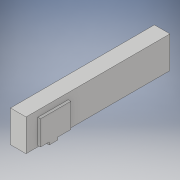
# Autodesk Inventor part: Nerf Gun
Saved by Autodesk Inventor 2018 (Build 220112000, 112)
## iProperties
Created: 2018-11-04
Part Number: Nerf Gun
Material: Generic
Document SubType Name: Modeling
Designer: Cameron
Density: 1 g/cm^3
Appearance: Default
Author: Cameron
Autodesk Inventor part; units mm, degrees
ref_plane "YZ Plane" through (0, 0, 0) normal (1, 0, 0) x (0, 1, 0)
ref_plane "XZ Plane" through (0, 0, 0) normal (0, 1, 0) x (-1, 0, 0)
ref_plane "XY Plane" through (0, 0, 0) normal (0, 0, 1) x (1, 0, 0)
sketch "Sketch1" plane through (0, 0, 0) normal (1, 0, 0) x (0, 1, 0)
  line L0 (42.5, 52.75) -> (-42.5, 52.75)
  line L1 (-42.5, 52.75) -> (-42.5, -52.75)
  line L2 (-42.5, -52.75) -> (42.5, -52.75)
  line L3 (42.5, -52.75) -> (42.5, 52.75)
  line L4 (-42.5, 22.75) -> (-51.5, 22.75)
  line L5 (-51.5, 22.75) -> (-51.5, -7.25)
  line L6 (-51.5, -7.25) -> (-42.5, -7.25)
  line L7 (-42.5, -7.25) -> (-42.5, 22.75)
  point P0 (0, 0)
  dimension "d0" = 105.5
  dimension "d1" = 85
  dimension "d2" = 42.5
  dimension "d3" = 52.75
  dimension "d4" = 30
  dimension "d5" = 30
  dimension "d6" = 9
  constraints: 16 end point, 4 parallel, 2 horizontal, 2 perpendicular, 1 point on line
  measures "d0" distance of L2.end L0.start
  measures "d1" distance of L0.start L0.end
  measures "d2" distance from line of point (0, 0) L3
  measures "d3" distance from line of point (0, 0) L0
  measures "d4" distance between parallel lines of L0 L4
  measures "d5" distance of L4.end L5.end
  measures "d6" distance between parallel lines of L1 L5
extrude "Extrusion1" add sketch "Sketch1" against normal blind 9
sketch "Sketch2" plane through (-9, 0, 0) normal (-1, 0, 0) x (0, 0, 1)
  point P0 (0, 0)
sketch "Sketch3" plane through (-9, 0, 0) normal (-1, 0, 0) x (0, 0, 1)
  line L0 (93.9, 64) -> (-406.1, 64)
  line L1 (-406.1, 64) -> (-406.1, -46.5)
  line L2 (-406.1, -46.5) -> (93.9, -46.5)
  line L3 (93.9, -46.5) -> (93.9, 64)
  line L4 (22.75, -51.5) -> (22.75, -42.5) projected
  line L5 (22.75, -42.5) -> (52.75, -42.5) projected
  line L6 (52.75, -42.5) -> (52.75, 42.5) projected
  line L7 (52.75, 42.5) -> (-52.75, 42.5) projected
  line L8 (-52.75, 42.5) -> (-52.75, -42.5) projected
  line L9 (-52.75, -42.5) -> (-7.25, -42.5) projected
  line L10 (-7.25, -42.5) -> (-7.25, -51.5) projected
  line L11 (-7.25, -51.5) -> (22.75, -51.5) projected
  point P0 (0, 0)
  dimension "d9" = 41.15
  dimension "d10" = 500
  dimension "d12" = 21.5
  dimension "d13" = 4
  constraints: 8 end point, 2 parallel, 1 horizontal, 1 perpendicular
  measures "d9" distance between parallel lines of L3 L6
  measures "d10" distance of L0.start L0.end
  measures "d12" distance between parallel lines of L0 L7
  measures "d13" distance between parallel lines of L5 L2
extrude "Extrusion2" add sketch "Sketch3" along normal blind 54 contours L3 L2 L4 L5 L6 L7 L8 L9 L10 L1 L0 | L2 L10 L9 L8 L7 L6 L5 L4
sketch "Sketch4" plane through (-63, 0, 0) normal (-1, 0, 0) x (0, 0, 1)
  line L0 (47.4, 22.73) -> (-47.5, 22.73)
  line L1 (-47.5, 22.73) -> (-47.5, 41)
  line L2 (-47.5, 41) -> (47.4, 41)
  line L3 (47.4, 41) -> (47.4, 22.73)
  line L4 (93.9, -46.5) -> (93.9, 64) projected
  line L5 (93.9, 64) -> (-406.1, 64) projected
  point P0 (0, 0)
  dimension "d16" = 46.5
  dimension "d17" = 23
  dimension "d18" = 94.9
  dimension "d19" = 18.27
  constraints: 8 end point, 2 parallel, 1 horizontal, 1 perpendicular
  measures "d16" distance between parallel lines of L4 L3
  measures "d17" distance between parallel lines of L5 L2
  measures "d18" distance of L0.start L0.end
  measures "d19" distance of L2.end L0.start
extrude "Extrusion3" add sketch "Sketch4" along normal blind 10.5
sketch "Sketch5" plane through (-63, 22.73, 47.4) normal (0, 0, 1) x (1, 0, 0)
  line L0 (-7.65, 18.27) -> (-4.25, 18.27)
  line L1 (-4.25, 18.27) -> (-4.25, 15.385)
  line L2 (-4.25, 15.385) -> (-7.65, 15.385)
  line L3 (-7.65, 15.385) -> (-7.65, 18.27)
  line L4 (-4.25, 2.885) -> (-7.65, 2.885)
  line L5 (-7.65, 2.885) -> (-7.65, 0)
  line L6 (-7.65, 0) -> (-4.25, 0)
  line L7 (-4.25, 0) -> (-4.25, 2.885)
  line L8 (0, 0) -> (-10.5, 0) projected
  line L9 (0, 18.27) -> (-10.5, 18.27) projected
  line L10 (-10.5, 0) -> (-10.5, 18.27) projected
  point P0 (63, -22.73)
  dimension "d22" = 12.5
  dimension "d23" = 0
  dimension "d24" = 0
  dimension "d26" = 2.885
  dimension "d27" = 2.85
  dimension "d28" = 2.885
  dimension "d29" = 3.4
  constraints: 16 end point, 4 parallel, 2 horizontal, 2 perpendicular, 2 point on line
  measures "d22" distance between parallel lines of L2 L4
  measures "d23" distance between parallel lines of L8 L6
  measures "d24" distance between parallel lines of L9 L0
  measures "d26" distance of L4.end L5.end
  measures "d27" distance between parallel lines of L10 L3
  measures "d28" distance between parallel lines of L0 L2
  measures "d29" distance of L1.end L2.end
extrude "Extrusion4" cut sketch "Sketch5" against normal blind 300
body "Solid1"
